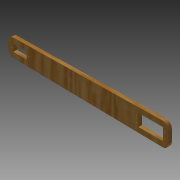
# Autodesk Inventor part: segment2a
Saved by Autodesk Inventor 2013 (Build 170138000, 138)
## iProperties
Created: 2014-10-09
Part Number: segment2a
Material: Plywood, Finish
Document SubType Name: Modeling
Designer: Masta
Density: 1 g/cm^3
Author: Masta
Autodesk Inventor part; units mm, degrees
ref_plane "YZ Plane" through (0, 0, 0) normal (1, 0, 0) x (0, 1, 0)
ref_plane "XZ Plane" through (0, 0, 0) normal (0, 1, 0) x (-1, 0, 0)
ref_plane "XY Plane" through (0, 0, 0) normal (0, 0, 1) x (1, 0, 0)
sketch "Sketch1" plane through (0, 0, 0) normal (0, 1, 0) x (-1, 0, 0)
  line L0 (0, 0) -> (31.5, 0)
  line L1 (223, -6) -> (246, -6)
  line L2 (246, -6) -> (246, 6)
  line L3 (246, 6) -> (223, 6)
  line L4 (223, 6) -> (223, -6)
  line L5 (223, -6) -> (246, 6) construction
  line L6 (246, -6) -> (223, 6) construction
  line L7 (234.5, 0) -> (248.5, 0) construction
  line L8 (234.5, 0) -> (220.5, 0) construction
  line L9 (0, 0) -> (18.5, 0) construction
  line L10 (223, 0) -> (240, 0) construction
  line L11 (0, 0) -> (-10.5, 0)
  line L12 (-20, 0) -> (-20, 20)
  line L13 (-20, 20) -> (255, 15)
  line L14 (255, 15) -> (255, 0)
  line L15 (255, 0) -> (240, 0) construction
  line L16 (255, 0) -> (246, 0)
  line L17 (-10.5, 10.5) -> (31.5, 10.5)
  line L18 (31.5, 10.5) -> (31.5, -10.5)
  line L19 (31.5, -10.5) -> (-10.5, -10.5)
  line L20 (-10.5, -10.5) -> (-10.5, 10.5)
  line L21 (-10.5, 10.5) -> (31.5, -10.5) construction
  line L22 (31.5, 10.5) -> (-10.5, -10.5) construction
  line L23 (-13.75, 5) -> (34.75, 5) construction
  line L24 (34.75, 5) -> (34.75, -5) construction
  line L25 (34.75, -5) -> (-13.75, -5) construction
  line L26 (-13.75, -5) -> (-13.75, 5) construction
  line L27 (-13.75, 5) -> (34.75, -5) construction
  line L28 (34.75, 5) -> (-13.75, -5) construction
  line L29 (31.5, 0) -> (223, 0)
  line L30 (-10.5, 0) -> (-20, 0)
  line L31 (-20, 0) -> (0, 0) construction
  point P0 (10.5, 0)
  point P1 (10.5, 0)
  dimension "d21" = 240
  dimension "d22" = 23
  dimension "d23" = 12
  dimension "d24" = 6
  dimension "d25" = 14
  dimension "d26" = 14
  dimension "d28" = 18.5
  dimension "d37" = 15
  dimension "d38" = 20
  dimension "d39" = 42
  dimension "d40" = 21
  dimension "d41" = 48.5
  dimension "d42" = 10
  dimension "d43" = 10.5
  constraints: 64 end point, 11 midpoint, 9 perpendicular, 7 parallel, 7 point on line, 6 coincident, 6 horizontal, 3 collinear
  measures "d21" distance of L0.start L10.end
  measures "d22" distance of L3.end L2.end
  measures "d23" distance of L2.end L1.end
  measures "d24" distance from line of L10.end L2
  measures "d25" distance of L7.start L7.end
  measures "d26" distance of L7.start L8.end
  measures "d28" distance of L0.start L9.end
  measures "d37" distance of L13.end L14.end
  measures "d38" distance of L12.start L12.end
  measures "d39" distance of L18.end L19.end
  measures "d40" distance of L17.end L18.end
  measures "d41" distance of L24.end L25.end
  measures "d42" distance of L23.end L24.end
  measures "d43" distance from line of L20 point (0, 0)
extrude "Extrusion1" add sketch "Sketch1" along normal blind 6 contours L18 L17 L20 L30 L12 L13 L14 L16 L2 L3 L4 L29
hole "Hole3" at (0, 0, 0) at (-248.5, 0, 0) at (-220.5, 0, 0) at (13.75, 0, 5) at (-34.75, 0, 5) direction (0, 1, 0) diameter 2 end through all
fillet "Fillet1" radius 10 2 edges at (-255, 3, 15) (20, 3, 20)
mirror "Mirror1" about plane through (-31.5, 0, 0) normal (0, 0, -1)
body "Solid1"
